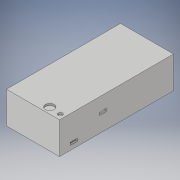
# Autodesk Inventor part: Pièce3
Saved by Autodesk Inventor 2019 (Build 230136000, 136)
## iProperties
Created: 2018-04-24
Part Number: Pièce3
Material: Générique
Document SubType Name: Modeling
Designer: Noah
Density: 1 g/cm^3
Appearance: Par défaut
Author: Noah
Autodesk Inventor part; units mm, degrees
ref_plane "YZ Plane" through (0, 0, 0) normal (1, 0, 0) x (0, 1, 0)
ref_plane "XZ Plane" through (0, 0, 0) normal (0, 1, 0) x (-1, 0, 0)
ref_plane "XY Plane" through (0, 0, 0) normal (0, 0, 1) x (1, 0, 0)
sketch "Esquisse1" plane through (0, 0, 0) normal (0, 1, 0) x (-1, 0, 0)
  line L0 (29.9796, 34.6939) -> (-26.0204, 34.6939)
  line L1 (-26.0204, 34.6939) -> (-26.0204, -50.3061)
  line L2 (29.9796, -50.3061) -> (29.9796, 34.6939)
  circle A0 centre (26.4796, 31.1939) radius 1.375
  circle A1 centre (-22.5204, 31.1939) radius 1.375
  circle A2 centre (26.4796, -26.8061) radius 1.375
  circle A3 centre (-22.5204, -26.8061) radius 1.375
  circle A4 centre (26.4796, 31.1939) radius 2.875
  circle A5 centre (-22.5204, 31.1939) radius 2.875
  circle A6 centre (-22.5204, -26.8061) radius 2.875
  circle A7 centre (26.4796, -26.8061) radius 2.875
  line L3 (-26.0204, -50.3061) -> (-26.0204, -90.3061)
  line L4 (-26.0204, -90.3061) -> (29.9796, -90.3061)
  line L5 (29.9796, -90.3061) -> (29.9796, -50.3061)
  line L6 (31.9796, 36.6939) -> (-28.0204, 36.6939)
  line L7 (-28.0204, 36.6939) -> (-28.0204, -92.3061)
  line L8 (-28.0204, -92.3061) -> (31.9796, -92.3061)
  line L9 (31.9796, -92.3061) -> (31.9796, 36.6939)
  point P0 (0, 0)
  dimension "d3" = 2.75
  dimension "d4" = 3.5
  dimension "d5" = 2.75
  dimension "d6" = 3.5
  dimension "d7" = 3.5
  dimension "d8" = 49
  dimension "d9" = 2.75
  dimension "d10" = 58
  dimension "d11" = 3.5
  dimension "d12" = 2.75
  dimension "d13" = 3.5
  dimension "d14" = 58
  dimension "d15" = 5.75
  dimension "d16" = 5.75
  dimension "d17" = 5.75
  dimension "d18" = 5.75
  dimension "d21" = 2
  dimension "d22" = 2
  dimension "d23" = 2
  dimension "d24" = 2
  dimension "d25" = 125
  constraints: 20 end point, 8 centre point, 4 coincident, 4 parallel, 2 horizontal, 2 perpendicular
  measures "d3" diameter of A0
  measures "d4" distance from line of A0.centre L0
  measures "d5" diameter of A1
  measures "d6" distance from line of A1.centre L1
  measures "d7" distance from line of L0 A1.centre
  measures "d8" distance of A0.centre A1.centre
  measures "d9" diameter of A2
  measures "d10" distance of A0.centre A2.centre
  measures "d11" distance from line of L2 A2.centre
  measures "d12" diameter of A3
  measures "d13" distance from line of L1 A3.centre
  measures "d14" distance of A1.centre A3.centre
  measures "d15" diameter of A4
  measures "d16" diameter of A5
  measures "d17" diameter of A6
  measures "d18" diameter of A7
  measures "d21" distance between parallel lines of L9 L5
  measures "d22" distance between parallel lines of L4 L8
  measures "d23" distance between parallel lines of L7 L3
  measures "d24" distance between parallel lines of L6 L0
  measures "d25" distance between parallel lines of L0 L4
extrude "Extrusion1" add sketch "Esquisse1" along normal blind 2 contours L2 L5 L4 L3 L1 L0 | L9 L8 L7 L6
sketch "Esquisse2" plane through (0, 0, 0) normal (0, -1, 0) x (1, 0, 0)
  circle A0 centre (22.5204, 31.1939) radius 2.875 projected
  circle A1 centre (22.5204, 31.1939) radius 1.375
  circle A2 centre (-26.4796, 31.1939) radius 1.375
  circle A3 centre (22.5204, -26.8061) radius 1.375
  circle A4 centre (-26.4796, -26.8061) radius 1.375
  circle A5 centre (22.5204, -26.8061) radius 2.875 projected
  circle A6 centre (-26.4796, -26.8061) radius 2.875 projected
  circle A7 centre (-26.4796, 31.1939) radius 2.875 projected
  point P0 (0, 0)
  dimension "d28" = 2.75
  dimension "d29" = 2.75
  dimension "d30" = 2.75
  dimension "d31" = 2.75
  dimension "d33" = 0
  dimension "d34" = 0
  dimension "d35" = 0
  dimension "d36" = 0
  dimension "d37" = 0
  constraints: 4 centre point, 1 coincident
  measures "d28" diameter of A1
  measures "d29" diameter of A2
  measures "d30" diameter of A3
  measures "d31" diameter of A4
  measures "d33" distance of A5.centre A3.centre
  measures "d34" distance of A5.centre A3.centre
  measures "d35" distance of A6.centre A4.centre
  measures "d36" distance of A6.centre A4.centre
  measures "d37" distance of A7.centre A2.centre
extrude "Extrusion2" add sketch "Esquisse2" against normal blind 4
sketch "Esquisse3" plane through (0, 2, 0) normal (0, 1, 0) x (1, 0, 0)
  line L0 (-29.9796, -34.6939) -> (26.0204, -34.6939)
  line L1 (26.0204, -34.6939) -> (26.0204, 90.3061)
  line L2 (26.0204, 90.3061) -> (-29.9796, 90.3061)
  line L3 (-29.9796, 90.3061) -> (-29.9796, -34.6939)
  line L4 (-31.9796, 92.3061) -> (-31.9796, -36.6939) projected
  line L5 (-31.9796, -36.6939) -> (28.0204, -36.6939) projected
  line L6 (28.0204, 92.3061) -> (-31.9796, 92.3061) projected
  line L7 (28.0204, -36.6939) -> (28.0204, 92.3061) projected
  point P0 (0, 0)
  dimension "d40" = 2
  dimension "d41" = 2
  dimension "d42" = 2
  dimension "d43" = 2
  constraints: 8 end point, 2 parallel, 1 horizontal, 1 perpendicular
  measures "d40" distance between parallel lines of L4 L3
  measures "d41" distance between parallel lines of L5 L0
  measures "d42" distance between parallel lines of L6 L2
  measures "d43" distance between parallel lines of L7 L1
extrude "Extrusion3" add sketch "Esquisse3" along normal blind 18
sketch "Esquisse4" plane through (28.0204, 0, -92.3061) normal (0, 0, -1) x (-1, 0, 0)
  line L0 (22, 20) -> (36, 20)
  line L1 (36, 20) -> (36, 5)
  line L2 (36, 5) -> (22, 5)
  line L3 (22, 5) -> (22, 20)
  line L4 (40, 20) -> (54, 20)
  line L5 (54, 20) -> (54, 5)
  line L6 (54, 5) -> (40, 5)
  line L7 (40, 5) -> (40, 20)
  line L8 (0, 0) -> (60, 0) projected
  line L9 (0, 0) -> (0, 20) projected
  point P0 (28.0204, 0)
  dimension "d46" = 5
  dimension "d47" = 5
  dimension "d48" = 14
  dimension "d49" = 14
  dimension "d51" = 22
  dimension "d52" = 40
  dimension "d53" = 15
  constraints: 16 end point, 4 parallel, 2 horizontal, 2 perpendicular, 1 point on line
  measures "d46" distance between parallel lines of L8 L6
  measures "d47" distance between parallel lines of L8 L2
  measures "d48" distance between parallel lines of L3 L1
  measures "d49" distance between parallel lines of L7 L5
  measures "d51" distance between parallel lines of L9 L3
  measures "d52" distance between parallel lines of L9 L7
  measures "d53" distance between parallel lines of L0 L2
extrude "Extrusion4" cut sketch "Esquisse4" against normal blind 20
sketch "Esquisse5" plane through (28.0204, 0, 36.6939) normal (1, 0, 0) x (0, 0, -1)
  line L0 (12, 8) -> (20, 8)
  line L1 (20, 8) -> (20, 5)
  line L2 (20, 5) -> (12, 5)
  line L3 (12, 5) -> (12, 8)
  line L4 (0, 0) -> (0, 20) projected
  line L5 (0, 0) -> (129, 0) projected
  point P0 (36.6939, 0)
  dimension "d56" = 12
  dimension "d57" = 8
  dimension "d58" = 3
  dimension "d59" = 5
  constraints: 8 end point, 2 parallel, 1 horizontal, 1 perpendicular
  measures "d56" distance between parallel lines of L3 L4
  measures "d57" distance between parallel lines of L3 L1
  measures "d58" distance between parallel lines of L0 L2
  measures "d59" distance between parallel lines of L5 L2
extrude "Extrusion5" cut sketch "Esquisse5" against normal blind 20
sketch "Esquisse6" plane through (28.0204, 0, 36.6939) normal (1, 0, 0) x (0, 0, -1)
  line L0 (53, 21) -> (45, 21)
  line L1 (45, 21) -> (45, 18)
  line L2 (45, 18) -> (53, 18)
  line L3 (53, 18) -> (53, 21)
  line L4 (0, 0) -> (129, 0) projected
  line L5 (0, 20) -> (129, 20) projected
  line L6 (0, 0) -> (0, 20) projected
  point P0 (36.6939, 0)
  dimension "d62" = 18
  dimension "d66" = 3
  dimension "d67" = 8
  dimension "d68" = 45
  constraints: 8 end point, 2 parallel, 1 horizontal, 1 perpendicular
  measures "d62" distance between parallel lines of L4 L2
  measures "d66" distance between parallel lines of L0 L2
  measures "d67" distance between parallel lines of L3 L1
  measures "d68" distance between parallel lines of L6 L1
sketch "Esquisse7" plane through (0, 20, 0) normal (0, 1, 0) x (1, 0, 0)
  line L0 (-31.9796, 92.3061) -> (-31.9796, -36.6939) projected
  line L1 (28.0204, 92.3061) -> (6.0204, 92.3061) projected
  line L2 (-31.9796, -36.6939) -> (28.0204, -36.6939)
  line L3 (28.0204, -36.6939) -> (28.0204, 92.3061)
  line L4 (28.0204, 92.3061) -> (-31.9796, 92.3061)
  line L5 (-31.9796, 92.3061) -> (-31.9796, -36.6939)
  line L6 (26.0204, 90.3061) -> (-29.9796, 90.3061) projected
  line L7 (26.0204, 90.3061) -> (26.0204, -34.6939) projected
  line L8 (-29.9796, 90.3061) -> (26.0204, 90.3061)
  line L9 (26.0204, 90.3061) -> (26.0204, -34.6939)
  line L10 (26.0204, -34.6939) -> (-29.9796, -34.6939)
  line L11 (-29.9796, -34.6939) -> (-29.9796, 90.3061)
  point P0 (0, 0)
  constraints: 16 end point, 4 parallel, 2 horizontal, 2 perpendicular
extrude "Extrusion6" add sketch "Esquisse7" along normal blind 14
extrude "Extrusion7" cut sketch "Esquisse6" against normal blind 14
sketch "Esquisse8" plane through (0, 34, 0) normal (0, 1, 0) x (1, 0, 0)
  line L0 (-31.9796, 92.3061) -> (-31.9796, -36.6939) projected
  line L1 (28.0204, -36.6939) -> (28.0204, 92.3061) projected
  line L2 (-31.9796, -36.6939) -> (28.0204, -36.6939)
  line L3 (28.0204, -36.6939) -> (28.0204, 92.3061)
  line L4 (28.0204, 92.3061) -> (-31.9796, 92.3061)
  line L5 (-31.9796, 92.3061) -> (-31.9796, -36.6939)
  point P0 (0, 0)
  constraints: 8 end point, 2 parallel, 1 horizontal, 1 perpendicular
extrude "Extrusion8" add sketch "Esquisse8" along normal blind 2
sketch "Esquisse9" plane through (0, 36, 0) normal (0, 1, 0) x (1, 0, 0)
  circle A0 centre (10.0204, -29.6939) radius 5
  line L0 (28.0204, -36.6939) -> (28.0204, 92.3061) projected
  line L1 (-31.9796, -36.6939) -> (28.0204, -36.6939) projected
  point P0 (0, 0)
  dimension "d75" = 10
  dimension "d76" = 18
  dimension "d77" = 7
  constraints: 1 centre point
  measures "d75" diameter of A0
  measures "d76" distance from line of L0 A0.centre
  measures "d77" distance from line of L1 A0.centre
extrude "Extrusion9" cut sketch "Esquisse9" against normal blind 3
sketch "Esquisse10" plane through (0, 36, 0) normal (0, 1, 0) x (1, 0, 0)
  circle A0 centre (23.0204, -30.6939) radius 2.5
  circle A1 centre (10.0204, -29.6939) radius 5 projected
  line L0 (-31.9796, -36.6939) -> (28.0204, -36.6939) projected
  point P0 (0, 0)
  dimension "d80" = 13
  dimension "d81" = 5
  dimension "d82" = 6
  constraints: 1 centre point
  measures "d80" horizontal distance of A1.centre A0.centre
  measures "d81" diameter of A0
  measures "d82" distance from line of L0 A0.centre
extrude "Extrusion10" cut sketch "Esquisse10" against normal blind 3 contours A0
